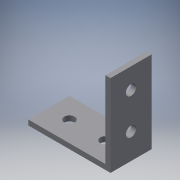
# Autodesk Inventor part: 2x1 angle bracket
Saved by Autodesk Inventor 2017 (Build 210142000, 142)
## iProperties
Created: 2016-10-10
Part Number: 2x1 angle bracket
Material: Aluminum 6061
Document SubType Name: Modeling
Designer: gus
Density: 2.7 g/cm^3
Appearance: Aluminum - Flat
Author: gus
Autodesk Inventor part; units mm, degrees
ref_plane "YZ Plane" through (0, 0, 0) normal (1, 0, 0) x (0, 1, 0)
ref_plane "XZ Plane" through (0, 0, 0) normal (0, 1, 0) x (-1, 0, 0)
ref_plane "XY Plane" through (0, 0, 0) normal (0, 0, 1) x (1, 0, 0)
sketch "Sketch1" plane through (0, 0, 0) normal (0, 0, 1) x (1, 0, 0)
  line L0 (0, 0) -> (-50.8, 0)
  line L1 (-50.8, 0) -> (-50.8, 3.175)
  line L2 (-50.8, 3.175) -> (-3.175, 3.175)
  line L3 (-3.175, 3.175) -> (-3.175, 50.8)
  line L4 (-3.175, 50.8) -> (0, 50.8)
  line L5 (0, 50.8) -> (0, 0)
  dimension "d0" = 3.175
  dimension "d1" = 50.8
  constraints: 12 end point, 7 perpendicular, 1 horizontal
  measures "d0" distance between parallel lines of L5 L3
  measures "d1" distance of L0.start L0.end
extrude "Extrusion1" add sketch "Sketch1" along normal blind 25.4
sketch "Sketch2" plane through (-50.8, 0, 0) normal (0, -1, 0) x (1, 0, 0)
  line L0 (50.8, 0) -> (50.8, 25.4) projected
  line L1 (0, 25.4) -> (50.8, 25.4) projected
  point P0 (12.7, 12.7)
  point P1 (34.925, 12.7)
  dimension "d4" = 15.875
  dimension "d5" = 22.225
  dimension "d6" = 12.7
  dimension "d7" = 12.7
  measures "d4" distance from line of L0 point (34.925, 12.7)
  measures "d5" distance of point (12.7, 12.7) point (34.925, 12.7)
  measures "d6" distance from line of L1 point (34.925, 12.7)
  measures "d7" distance from line of L1 point (12.7, 12.7)
hole "Hole1" at (-38.1, 0, 12.7) at (-15.875, 0, 12.7) direction (0, 1, 0) diameter 6.35 end through all
sketch "Sketch3" plane through (0, 0, 0) normal (1, 0, 0) x (0, 0, -1)
  line L0 (0, 50.8) -> (0, 0) projected
  line L1 (-15.875, 3.175) -> (-9.525, 3.175) projected
  point P0 (-12.7, 15.875)
  point P1 (-12.7, 38.1)
  dimension "d15" = 12.7
  dimension "d16" = 12.7
  dimension "d17" = 12.7
  dimension "d18" = 22.225
  measures "d15" distance from line of L0 point (-12.7, 38.1)
  measures "d16" distance from line of L0 point (-12.7, 15.875)
  measures "d17" distance from line of L1 point (-12.7, 15.875)
  measures "d18" distance of point (-12.7, 38.1) point (-12.7, 15.875)
hole "Hole2" at (0, 15.875, 12.7) at (0, 38.1, 12.7) direction (-1, 0, 0) diameter 6.35 end through all
body "Solid1"
